Autodesk Fusion 360 part; units mm, degrees
(part 3 of 3)
extrude "Extrusion1" add sketch "Skizze1" against normal blind 0.5 makes body 1 at (-70, -32.1561, 133.405) makes body 2 at (-70, -60.7536, 132.9413) makes body 3 at (-70, -57.1892, 114.2352) makes body 4 at (-70, 22.312, 115.3036) makes body 5 at (-70, -20.911, 115.4779) makes body 6 at (-70, 51.7894, 115.6413) makes body 7 at (-70, 1.4786, 115.2044) makes body 8 at (-70, 6.1695, 97.5534) makes body 9 at (-70, 1.7117, 133.9952) makes body 10 at (-70, 11.2349, 97.2549) makes body 11 at (-70, -1.5466, 114.6098) makes body 12 at (-70, 46.6405, 147.5925) makes body 13 at (-70, 14.8553, 132.5243) makes body 14 at (-70, -7.0834, 115.2044) makes body 15 at (-70, -24.7061, 96.2352) makes body 16 at (-70, 63.5119, 116.2668) makes body 17 at (-70, -58.7866, 115.2549) makes body 18 at (-70, -26.3034, 97.2549) makes body 19 at (-70, 47.7927, 113.5062) makes body 20 at (-70, -26.3251, 133.405) makes body 21 at (-70, -66.3226, 132.8319) makes body 22 at (-70, -25.932, 115.405) makes body 23 at (-70, 4.8997, 114.8285) makes body 24 at (-70, 12.8323, 96.2352) makes body 25 at (-70, -31.7631, 115.405) makes body 26 at (-70, -54.476, 133.0929) makes body 27 at (-70, 57.9562, 147.7668) makes body 28 at (-70, -2.6155, 132.6098) makes body 29 at (-70, 63.0114, 147.7668) makes body 30 at (-70, 15.5786, 114.5243) makes body 31 at (-70, -38.5682, 112.7174) makes body 32 at (-70, 58.4567, 116.2668) makes body 33 at (-70, -61.6178, 89.8475) makes body 34 at (-70, -63.852, 115.5534) makes body 35 at (-70, -21.3041, 133.4779) makes body 36 at (-70, 3.8308, 132.8285) makes body 37 at (-70, 21.5887, 133.3036) makes body 38 at (-70, 51.2889, 147.1413) makes body 39 at (-70, -39.613, 133.3036) makes body 40 at (-70, 18.3473, 130.7174) makes body 41 at (-70, 25.1947, 132.7431) makes body 42 at (-70, -31.3689, 97.5534) makes body 43 at (-70, 26.0558, 114.3967) makes body 44 at (-70, 19.0707, 112.7174)
